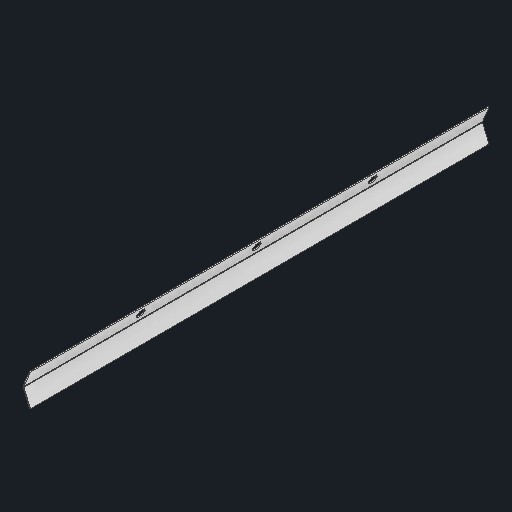
# Autodesk Inventor part: DMF 01 17 опора крышки v2.1_CPY
Saved by Autodesk Inventor 2026.2 (Build 302298010, 298A)
## iProperties
Created: 2024-04-30
Part Number: DMF 01 17 опора крышки v2.1_CPY
Material: Stainless Steel AISI 304
Document SubType Name: Sheet Metal
Designer: pokla
Stock Number: Барабан_Полка_Крышки
Density: 8 g/cm^3
Flat Pattern Width: 7.47819 cm
Flat Pattern Length: 98.85 cm
Flat Pattern Area: 739.22 cm^2
Sheet Metal Rule: Default
Sheet Metal Width: 74,782 mm
Sheet Metal Length: 988,500 mm
Sheet Metal Area: 73921,954 mm^2
Appearance: Chrome - Satin
Author: pokla
Autodesk Inventor part; units mm, degrees
note: some values were not read from the file. Chosen so that the rebuilt part matches the saved one: flange form of "Plate3".
ref_plane "YZ Plane" through (0, 0, 0) normal (1, 0, 0) x (0, 1, 0)
ref_plane "XZ Plane" through (0, 0, 0) normal (0, 1, 0) x (-1, 0, 0)
ref_plane "XY Plane" through (0, 0, 0) normal (0, 0, 1) x (1, 0, 0)
sketch "Sketch4" plane through (0, 0, 0) normal (0, 0, 1) x (1, 0, 0)
  line L0 (-202.056852, 202.056852) -> (0, 285.751541) construction
  line L1 (0, 285.751541) -> (202.056852, 202.056852) construction
  line L2 (202.056852, 202.056852) -> (285.751541, 0) construction
  line L3 (285.751541, 0) -> (202.056852, -202.056852) construction
  line L4 (202.056852, -202.056852) -> (0, -285.751541) construction
  line L5 (0, -285.751541) -> (-202.056852, -202.056852) construction
  line L6 (-202.056852, -202.056852) -> (-285.751541, 0) construction
  line L7 (-285.751541, 0) -> (-202.056852, 202.056852) construction
  line L8 (-285.11749, 1.530734) -> (-271.241389, 35.030606)
  line L9 (-285.11749, -1.530734) -> (-271.241389, -35.030606)
  arc A0 (-285.11749, 1.530734) -> (-285.11749, -1.530734) centre (-281.421972, 0) ccw
  point P0 (0, 0)
  point P1 (0, 0)
  point P2 (0, 0)
  dimension "d16" = 528
  dimension "d23" = 36.26
  dimension "d24" = 4
  measures "d16" distance between parallel lines of L7 L3
  measures "d23" distance of L8.start L8.end
  measures "d24" radius of A0
contour flange "Contour Flange1" sketch "Sketch4" thickness 2 bend radius 2 width 988.5 along (0, 0, -1) mid plane no both sides no wall seen from (-278.17944, 18.28067, 0) lies toward (0.9238795, -0.3826834, 0) curves L8 A0 L9
bend "Bend2"
corner "Corner2"
sketch "Sketch6" plane through (-285.11749, 1.530734, 0) normal (-0.9238795, 0.3826834, 0) x (0.3826834, 0.9238795, 0)
  circle A0 centre (19.22, 40.75) radius 5.5 construction
  circle A1 centre (19.22, 947.75) radius 5.5 construction
  line L0 (0, 0) -> (0, 988.5)
  line L1 (36.26, 988.5) -> (0, 988.5)
  line L2 (36.26, 0) -> (0, 0)
  line L3 (27.62, 942.900258) -> (19.22, 938.050515)
  line L4 (19.22, 938.050515) -> (10.82, 942.900258)
  line L5 (10.82, 942.900258) -> (10.82, 952.599742)
  line L6 (10.82, 952.599742) -> (19.22, 957.449485)
  line L7 (19.22, 957.449485) -> (27.62, 952.599742)
  line L8 (27.62, 952.599742) -> (27.62, 942.900258)
  line L9 (27.62, 35.900258) -> (19.22, 31.050515)
  line L10 (19.22, 31.050515) -> (10.82, 35.900258)
  line L11 (10.82, 35.900258) -> (10.82, 45.599742)
  line L12 (10.82, 45.599742) -> (19.22, 50.449485)
  line L13 (19.22, 50.449485) -> (27.62, 45.599742)
  line L14 (27.62, 45.599742) -> (27.62, 35.900258)
  point P0 (107.695526, 0)
  dimension "d36" = 11
  dimension "d41" = 11
  dimension "d93" = 19.22
  dimension "d94" = 40.75
  dimension "d95" = 19.22
  dimension "d96" = 40.75
  dimension "d98" = 16.8
  dimension "d99" = 16.8
  constraints: 24 end point, 2 centre point, 2 coincident, 2 parallel, 26 other
  measures "d36" diameter of A0
  measures "d41" diameter of A1
  measures "d93" distance from line of L0 A0.centre
  measures "d94" distance from line of L2 A0.centre
  measures "d95" distance from line of L0 A1.centre
  measures "d96" distance from line of L1 A1.centre
  measures "d98" distance between parallel lines of L6 L3
  measures "d99" distance between parallel lines of L12 L9
extrude "Extrusion1" [suppressed]
sketch "Sketch13" plane through (-285.11749, 1.530734, 0) normal (-0.9238795, 0.3826834, 0) x (0.3826834, 0.9238795, 0)
  circle A0 centre (19.22, 494.25) radius 5.5 construction
  line L0 (36.26, 0) -> (36.26, 988.5)
  line L1 (36.26, 0) -> (0, 0)
  line L2 (27.62, 489.400258) -> (19.22, 484.550515)
  line L3 (19.22, 484.550515) -> (10.82, 489.400258)
  line L4 (10.82, 489.400258) -> (10.82, 499.099742)
  line L5 (10.82, 499.099742) -> (19.22, 503.949485)
  line L6 (19.22, 503.949485) -> (27.62, 499.099742)
  line L7 (27.62, 499.099742) -> (27.62, 489.400258)
  point P0 (107.695526, 0)
  point P1 (36.26, 494.25)
  point P2 (35, 910)
  point P3 (35, 1110)
  point P4 (18.13, 0)
  point P5 (27.62, 494.25)
  dimension "d83" = 11
  dimension "magic_d1" = 17.04
  dimension "d97" = 16.8
  constraints: 12 end point, 2 horizontal alignment, 2 midpoint, 1 centre point, 1 coincident, 15 other
  measures "d83" diameter of A0
  measures "d97" distance between parallel lines of L4 L7
extrude "Extrusion7" cut sketch "Sketch13" against normal through all
pattern_linear "Rectangular Pattern5" count 3 spacing 250 along (0, 0, 1) of "Extrusion7" first direction both ways yes
equation "\"d16\" = Барабан_размер_по_плоскостям - Thickness"
equation "\"d24\" = BendRadius + Thickness"
equation "\"d41\" = d36"
equation "\"d95\" = d93"
equation "\"d96\" = d94"
equation "\"d99\" = d98"
equation "\"d25\" = Thickness"
equation "\"d26\" = BendReliefWidth"
equation "\"d27\" = BendReliefDepth"
equation "\"d28\" = MinimumRemnant"
equation "\"d29\" = TransitionRadius"
equation "\"d31\" = BendRadius"
equation "\"d33\" = CornerReliefSize"
equation "\"d34\" = GapSize"
equation "\"d35\" = JacobiRadiusSize"
equation "\"BendRadius\" = Thickness"
equation "\"BendReliefWidth\" = Thickness"
equation "\"BendReliefDepth\" = 0.5 * Thickness"
equation "\"CornerReliefSize\" = 4 * Thickness"
equation "\"MinimumRemnant\" = 2 * Thickness"
equation "\"TransitionRadius\" = BendRadius"
equation "\"JacobiRadiusSize\" = BendRadius"
equation "\"GapSize\" = Thickness"
equation "\"Барабан_размер_по_плоскостям\" = 530"
equation "\"Thickness\" = 2"
body "Solid2"
